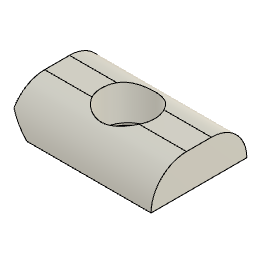
Slide-in Nut Support (Autodesk Fusion 360 design; units mm, degrees)
Autodesk Fusion 360 part; units mm, degrees
sketch "Sketch1" plane through (0, 0, 0) normal (0, 0, 1) x (1, 0, 0)
  line L0 (4, 2.7) -> (-4, 2.7)
  line L1 (-4, 2.7) -> (-4, -2.7)
  line L2 (-4, -2.7) -> (4, -2.7)
  line L3 (4, -2.7) -> (4, 2.7)
  line L4 (4, 2.7) -> (-4, -2.7) construction
  line L5 (-4, 2.7) -> (4, -2.7) construction
  circle A0 centre (0, 0) radius 1.5
  dimension "d1" = 5.4
  dimension "d2" = 8
  dimension "d3" = 3
  constraint horizontal L0
  constraint perpendicular L0 L1
  constraint parallel L0 L2
  constraint parallel L1 L3
  constraint coincident L4 A0.centre
  constraint coincident L5 A0.centre
  constraint coincident A0.centre origin
  constraint midpoint L5 A0.centre
  measures "d1" distance of L0.end L1.end
  measures "d2" distance of L0.start L0.end
  measures "d3" diameter of A0
extrude "Extrude1" add sketch "Sketch1" along normal blind 2.4
fillet "Fillet1" radius 2 2 edges at (0, -2.7, 2.4) (0, 2.7, 2.4)
chamfer "Chamfer2" distance 1.4 distance2 1.4 1 edges at (-4, 0, 0) measured on face at (-4, 0.2333, 0.8)
sketch "Sketch2" plane through (0, 0, 0) normal (0, 0, -1) x (1, 0, 0)
  line L0 (-2.6, 2.7) -> (-2.6, -2.7)
  line L1 (-2.6, -2.7) -> (4, -2.7)
  line L2 (4, -2.7) -> (4, 2.7)
  line L3 (4, 2.7) -> (-2.6, 2.7)
  circle A0 centre (0, 0) radius 1.5
  line L4 (0, 2.7) -> (0, -2.7) construction
  line L5 (2.7, -2.7) -> (2.7, 2.7)
  dimension "d12" = 2.7
  constraint coincident L3 L4.start
  constraint coincident L1 L4.end
  constraint perpendicular L1 L4
  constraint coincident L1 L5.start
  constraint coincident L3 L5.end
  constraint perpendicular L3 L5
  constraint coincident A0.centre L4
  measures "d12" distance of L4.start L5.end
chamfer "Chamfer3" distance 0.4 angle 45 4 edges at (0.7, -2.7, 0) (4, 0, 0) (0.7, 2.7, 0) (-1.3985, 0.5424, 0)
equation "d12 = ( 5.4 / 2 ) * 1 mm"
